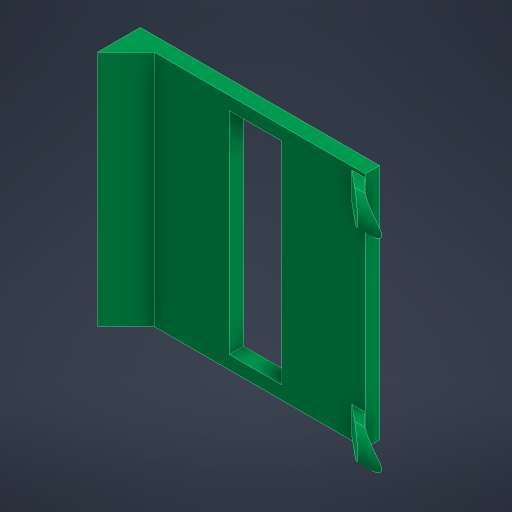
# Autodesk Inventor part: Cover Side (Normal)
Saved by Autodesk Inventor 2023.4 (Build 274418000, 418)
## iProperties
Created: 2023-02-07
Part Number: Cover Side (Normal)
Material: Generic
Document SubType Name: Modeling
Designer: xSibe
Density: 1 g/cm^3
Appearance: Plastic Dark Green
Author: xSibe
Autodesk Inventor part; units mm, degrees
ref_plane "YZ Plane" through (0, 0, 0) normal (1, 0, 0) x (0, 1, 0)
ref_plane "XZ Plane" through (0, 0, 0) normal (0, 1, 0) x (-1, 0, 0)
ref_plane "XY Plane" through (0, 0, 0) normal (0, 0, 1) x (1, 0, 0)
sketch "Sketch1" plane through (0, 0, 0) normal (0, 1, 0) x (-1, 0, 0)
  line L0 (-42.1, -24.9) -> (-7.7, -24.9)
  line L1 (-7.7, -22.55) -> (-7.7, -24.9)
  line L2 (-7.7, -22.55) -> (-42.1, -22.55)
  line L3 (-42.1, -22.55) -> (-42.1, -24.9)
  line L4 (-7.85, -24.75) -> (-41.95, -24.75)
  line L5 (-41.95, -24.75) -> (-41.95, -22.7)
  line L6 (-41.95, -22.7) -> (-7.85, -22.7)
  line L7 (-7.85, -22.7) -> (-7.85, -24.75)
  line L8 (-7.85, -22.7) -> (-11.85, -22.7)
  line L9 (-11.85, -22.7) -> (-11.85, -22.7)
  line L10 (-7.85, -18.7) -> (-7.85, -18.7)
  line L11 (-7.85, -18.7) -> (-7.85, -22.7)
  line L12 (-11.85, -22.7) -> (-7.85, -18.7)
  line L13 (0, -22.875) -> (0, -18.725)
  line L14 (-7.7, -22.875) -> (-7.7, -18.725)
  line L15 (-41.95, -22.7) -> (-39.95, -22.7)
  line L16 (-39.95, -22.7) -> (-39.95, -22.7)
  line L17 (-41.95, -20.7) -> (-41.95, -20.7)
  line L18 (-41.95, -20.7) -> (-41.95, -22.7)
  line L19 (-39.95, -22.7) -> (-41.95, -20.7)
  line L20 (-41.95, -20.7) -> (-44.07132, -18.57868)
  line L21 (-44.07132, -18.57868) -> (-45.97132, -18.57868)
  line L22 (-45.97132, -18.57868) -> (-41.95, -22.6)
  line L23 (-41.95, -22.6) -> (-39.8, -24.75)
  line L24 (-45.97132, -18.57868) -> (-45.02132, -17.62868)
  line L25 (-45.97132, -18.57868) -> (-44.198589, -18.57868) construction
  line L26 (-44.07132, -18.57868) -> (-45.02132, -17.62868)
  line L27 (-41.85, -24.825) -> (-41.85, -22.518934)
  point P0 (0, 0)
  point P1 (-11.85, -18.7)
  point P2 (-39.95, -20.7)
  point P3 (-7.85, -18.7)
  point P4 (-39.95, -22.7)
  point P5 (-41.95, -22.55)
  point P6 (-42, -22.55)
  point P7 (-41.85, -22.7)
  point P8 (-41.85, -24.75)
  dimension "d0" = 0.15
  dimension "d1" = 4
  dimension "d2" = 4
  dimension "d3" = 4
  dimension "d4" = 4
  dimension "d5" = 2
  dimension "d6" = 2
  dimension "d7" = 2
  dimension "d8" = 2
  dimension "d9" = 3
  dimension "d10" = 1.9
  dimension "d11" = 45
  dimension "d28" = 45
  constraints: 44 end point, 9 point on line, 4 horizontal, 4 parallel, 3 perpendicular, 1 collinear, 1 vertical, 5 other
  measures "d0" distance between parallel lines of L0 L4
  measures "d1" distance of point (-11.85, -18.7) L10.end
  measures "d2" distance of L8.end point (-11.85, -18.7)
  measures "d3" distance of L9.end point (-11.85, -18.7)
  measures "d4" distance of L10.start point (-11.85, -18.7)
  measures "d5" distance of L17.end point (-39.95, -20.7)
  measures "d6" distance of point (-39.95, -20.7) L15.end
  measures "d7" distance of L16.end point (-39.95, -20.7)
  measures "d8" distance of L17.start point (-39.95, -20.7)
  measures "d9" distance of L20.start L20.end
  measures "d10" distance of L20.end L21.end
  measures "d11" angle of L22 L21
  measures "d28" angle of L25 L24
extrude "Extrusion1" add sketch "Sketch1" along normal mid plane 33.75 contours L22 L21 L20 L18 L2 | L2 L18 L22 | L18 L19 L2 | L2 L27 L23 L18 | L24 L26 L21 | L11 L6 L12 L2 | L2 L12 L11 | L2 L19 L6 L27 | L6 L7 L4 L23 | L23 L4 L27
sketch "Sketch2" plane through (0, 0, 0) normal (0, 1, 0) x (-1, 0, 0)
  line L0 (-7.85, -24.75) -> (-41.85, -24.75)
  line L1 (-41.85, -22.7) -> (-45.97132, -18.57868)
  line L2 (-39.95, -22.7) -> (-11.85, -22.7)
  line L3 (-11.85, -22.7) -> (-7.85, -18.7)
  line L4 (-7.85, -18.7) -> (-7.85, -24.75)
  line L5 (-49.8, -18.72125) -> (-49.8, -22.87875)
  line L6 (-42.1, -22.55) -> (-45.92875, -18.72125)
  line L7 (0, -22.875) -> (0, -18.725)
  line L8 (-7.7, -22.875) -> (-7.7, -18.725)
  line L9 (-7.7, -18.725) -> (-7.85, -18.725)
  line L10 (-7.85, -18.725) -> (-7.85, -22.875)
  line L11 (-7.85, -22.875) -> (-7.7, -22.875)
  line L12 (-7.7, -22.875) -> (-7.7, -18.725)
  line L13 (-7.85, -18.725) -> (-6.35, -18.725)
  line L14 (-6.35, -18.725) -> (-6.35, -22.875)
  line L15 (-6.35, -22.875) -> (-7.85, -22.875)
  line L16 (-7.85, -22.875) -> (-7.85, -18.725)
  line L17 (-7.85, -22.725) -> (-6.5, -22.725)
  line L18 (-6.5, -22.725) -> (-6.5, -18.875)
  line L19 (-6.5, -18.875) -> (-7.85, -18.875)
  line L20 (-42.1, -22.87875) -> (-42.1, -22.55)
  line L21 (-42.1, -22.87875) -> (-41.67125, -22.87875)
  line L22 (-41.67125, -22.87875) -> (-42.67125, -22.87875)
  line L23 (-45.92875, -18.72125) -> (-45.82875, -18.72125)
  line L24 (-45.82875, -18.72125) -> (-48.32875, -18.72125)
  line L25 (-48.32875, -18.72125) -> (-42.67125, -22.87875)
  line L26 (-45.82875, -18.79625) -> (-48.100037, -18.79625)
  line L27 (-48.100037, -18.79625) -> (-42.646656, -22.80375)
  line L28 (-42.646656, -22.80375) -> (-41.67125, -22.80375)
  line L29 (-45.82875, -18.79625) -> (-45.75375, -18.79625)
  line L30 (-45.97132, -18.57868) -> (-45.02132, -17.62868)
  line L31 (-45.02132, -17.62868) -> (-39.95, -22.7)
  line L32 (-41.85, -24.75) -> (-41.85, -22.7)
  point P0 (0, 0)
  point P1 (-7.85, -18.875)
  point P2 (-41.74625, -22.80375)
  point P3 (-41.85, -22.80375)
  dimension "d17" = 1.5
  dimension "d18" = 0.15
  dimension "d22" = 1
  dimension "d23" = 2.5
  dimension "d24" = 0.075
  constraints: 42 end point, 8 point on line, 5 horizontal, 5 parallel, 3 perpendicular, 1 vertical, 6 other
  measures "d17" distance of L10.end L14.end
  measures "d18" distance between parallel lines of L14 L18
  measures "d22" distance of L21.end L22.end
  measures "d23" distance of L23.end L24.end
  measures "d24" distance between parallel lines of L24 L26
ref_plane "Work Plane2" through (0, -14.4, -20.8) normal (0, -1, 0) x (0, 0, -1)
ref_plane "Work Plane1" through (0, -24.9, 24.9) normal (0, -1, 0) x (0, 0, -1)
extrude "Extrusion2" add sketch "Sketch2" along normal mid plane 4 from surface at -14.4 contours L4 L19 L8 L17 | L28 L20 L6 L26 L29 L1 L32 | L8 L19 L18 L17 | L28 L27 L26 L6 L20
fillet "Fillet1" radius 2 10 edges at (7.175, -12.4, -18.875) (7.175, -16.4, -18.875) (7.175, -16.4, -22.725) (7.175, -12.4, -22.725) (45.7912, -12.4, -18.7963) (46.9644, -12.4, -18.7962) (46.9644, -16.4, -18.7962) (45.7912, -16.4, -18.7963) (42.2483, -16.4, -22.8038) (42.2483, -12.4, -22.8038)
sketch "Sketch3" plane through (46.04632, 0, -18.50368) normal (0, 1, 0) x (0.7071068, 0, -0.7071068)
  line L0 (0, 5.934493) -> (0, 0.106066)
  line L1 (0, 0.106066) -> (-1.343503, 0.106066)
  line L2 (-1.343503, 0.106066) -> (-1.343503, 7.277996)
  line L3 (-1.343503, 7.277996) -> (-21.213203, 27.147697)
  line L4 (-21.213203, 27.147697) -> (-26.870058, 27.147697)
  line L5 (-26.870058, 27.147697) -> (-22.592062, 31.425693)
  line L6 (-22.592062, 31.425693) -> (1.449569, 7.384062)
  line L7 (1.148836, 2.093348) -> (1.148836, 2.093348)
  line L8 (1.148836, 2.093348) -> (0, 3.242184)
  line L9 (0, 3.242184) -> (0, 3.242184)
  line L10 (0, 3.242184) -> (1.148836, 2.093348)
  line L11 (1.146923, 2.105868) -> (1.146923, 2.105868)
  line L12 (1.146923, 2.105868) -> (0, 3.252791)
  line L13 (0, 3.252791) -> (0, 5.934493)
  line L14 (0, 3.252791) -> (1.146923, 2.105868)
  line L15 (1.146923, 2.105868) -> (0, 3.252791)
  line L16 (1.148836, 2.093348) -> (1.146923, 2.105868)
  line L17 (0, 3.242184) -> (1.148836, 2.093348)
  line L18 (0, 3.252791) -> (0, 3.242184)
  line L19 (-25.3321, 28.685654) -> (-25.3321, 28.685654)
  line L20 (-24.023953, 30.099867) -> (-26.039207, 30.099867)
  line L21 (-24.023953, 30.099867) -> (-22.008699, 30.099867) construction
  line L22 (-26.85238, 27.27144) -> (-26.85238, 29.286695)
  line L23 (-26.85238, 27.27144) -> (-24.837126, 27.27144) construction
  line L24 (-27.860007, 28.279067) -> (-26.85238, 27.27144)
  line L25 (-25.03158, 31.107495) -> (-24.023953, 30.099867)
  line L26 (0.636683, 5.444535) -> (0.073362, 6.007855)
  line L27 (0.073362, 6.007855) -> (0.829619, 4.18209)
  line L28 (0.073362, 6.007855) -> (2.049557, 6.007855) construction
  line L29 (0.636683, 5.444535) -> (1.146923, 2.105868)
  line L30 (1.148836, 2.093348) -> (1.659075, -1.245318)
  line L31 (1.659075, -1.245318) -> (0.073362, 6.007855)
  line L32 (0, 0.413757) -> (0, 3.242184)
  line L33 (0, 0.413757) -> (-1.343503, 7.277996)
  line L34 (-0.671751, 0.106066) -> (-1.343503, 7.277996)
  line L35 (-26.286695, 29.640248) -> (-26.286695, 29.640248)
  line L36 (-26.286695, 29.640248) -> (-25.3321, 28.685654)
  line L37 (-25.3321, 28.685654) -> (-26.286695, 29.640248)
  line L38 (-27.700908, 28.226034) -> (-26.746314, 27.27144)
  line L39 (-27.700908, 28.226034) -> (-26.286695, 29.640248)
  line L40 (-26.286695, 29.640248) -> (-24.978547, 30.948396)
  line L41 (-24.978547, 30.948396) -> (-24.023953, 29.993801)
  line L42 (0, 5.934493) -> (1.659075, -1.245318)
  line L43 (0, 5.934493) -> (0, 5.934493)
  line L44 (0, 3.252791) -> (0, 5.934493)
  line L45 (1.449569, 7.384062) -> (0, 5.934493)
  point P0 (0.864735, 2.388056)
  point P1 (0.867703, 2.374481)
  point P2 (1.146923, 2.105868)
  point P3 (-24.130019, 30.099867)
  point P4 (-25.827075, 30.099867)
  point P5 (-26.85238, 29.074563)
  point P6 (-26.85238, 27.377506)
  dimension "d37" = 180
  dimension "d38" = 90
  dimension "d39" = 67.5
  constraints: 24 end point, 3 equal length, 3 horizontal, 1 midpoint, 1 perpendicular, 1 point on line, 1 other
  measures "d37" angle of L20 L21
  measures "d38" angle of L23 L22
  measures "d39" angle of L27 L28
extrude "Extrusion3" cut sketch "Sketch3" along normal mid plane 5 from surface at -14.4 contours L26 L29 L27 | L27 L29 L12 L31 | L12 L16 L8 L31 | L8 L30 L31
mirror "Mirror1" about plane through (0, 0, 0) normal (0, 1, 0) of "Extrusion2", "Fillet1", "Extrusion3"
extrude "Extrusion5" cut sketch "Sketch3" along normal mid plane 50 contours L34 L1 L2
sketch "Sketch5" plane through (41.95, 16.875, -24.75) normal (0, 0, -1) x (-1, 0, 0)
  line L0 (34.1, -33.75) -> (34.1, 0) projected
  line L1 (0.1, 0) -> (34.1, 0) projected
  line L2 (34.1, -33.75) -> (0.1, -33.75) projected
  line L3 (34.1, -16.875) -> (15.7, -16.875)
  line L4 (19.45, -31.875) -> (11.95, -31.875)
  line L5 (11.95, -31.875) -> (11.95, -1.875)
  line L6 (11.95, -1.875) -> (19.45, -1.875)
  line L7 (19.45, -1.875) -> (19.45, -31.875)
  line L8 (19.45, -31.875) -> (11.95, -1.875) construction
  line L9 (11.95, -31.875) -> (19.45, -1.875) construction
  line L10 (0.1, -33.75) -> (0.1, 0) projected
  point P0 (41.95, -16.875)
  dimension "d42" = 18.4
  dimension "d43" = 7.5
  dimension "d44" = 30
  constraints: 14 end point, 3 midpoint, 2 horizontal, 2 parallel, 1 perpendicular
  measures "d42" distance of L3.start L3.end
  measures "d43" distance of L5.end L6.end
  measures "d44" distance of L4.end L5.end
extrude "Extrusion6" cut sketch "Sketch5" against normal up to surface (2.05 mm away) contours L4 L5 L6 L7
sketch "Sketch6" plane through (41.85, 0, 0) normal (1, 0, 0) x (0, 1, 0)
  arc A0 (13.764204, -22.7) -> (14.4, -22.80375) centre (14.4, -20.80375) ccw
  line L0 (-13.764204, -22.7) -> (13.764204, -22.7)
  arc A1 (-14.4, -22.80375) -> (-13.764204, -22.7) centre (-14.4, -20.80375) ccw
  arc A2 (-15.035796, -22.7) -> (-14.4, -22.80375) centre (-14.4, -20.80375) ccw
  line L1 (-15.035796, -22.7) -> (-16.875, -22.7)
  line L2 (-16.875, -24.75) -> (-16.875, -22.7)
  line L3 (-16.875, -24.75) -> (16.875, -24.75)
  line L4 (16.875, -22.7) -> (16.875, -24.75)
  line L5 (15.035796, -22.7) -> (16.875, -22.7)
  arc A3 (14.4, -22.80375) -> (15.035796, -22.7) centre (14.4, -20.80375) ccw
  line L6 (16.875, -18.10368) -> (-16.875, -18.10368)
  arc A4 (16.4, -20.79625) -> (12.4, -20.79625) centre (14.4, -20.79625) ccw
  line L7 (12.4, -20.80375) -> (12.4, -20.79625)
  arc A5 (12.4, -20.80375) -> (14.4, -22.80375) centre (14.4, -20.80375) ccw
  arc A6 (14.4, -22.80375) -> (16.4, -20.80375) centre (14.4, -20.80375) ccw
  line L8 (16.4, -20.79625) -> (16.4, -20.80375)
  arc A7 (-12.4, -20.79625) -> (-16.4, -20.79625) centre (-14.4, -20.79625) ccw
  line L9 (-16.4, -20.80375) -> (-16.4, -20.79625)
  arc A8 (-16.4, -20.80375) -> (-14.4, -22.80375) centre (-14.4, -20.80375) ccw
  arc A9 (-14.4, -22.80375) -> (-12.4, -20.80375) centre (-14.4, -20.80375) ccw
  line L10 (-12.4, -20.79625) -> (-12.4, -20.80375)
  line L11 (14.4, -18.79625) -> (-14.4, -18.79625)
  line L12 (-16.875, -18.57868) -> (-16.875, -18.10368)
  line L13 (-16.875, -22.7) -> (-16.875, -18.57868)
  line L14 (16.875, -18.10368) -> (16.875, -18.57868)
  line L15 (16.875, -18.57868) -> (16.875, -22.7)
  line L16 (16.4, -20.80375) -> (16.4, -22.7)
  line L17 (-16.4, -20.80375) -> (-16.4, -22.7)
  line L18 (12.4, -20.80375) -> (12.4, -22.7)
  line L19 (-12.4, -20.80375) -> (-12.4, -22.7)
  point P0 (-15.035796, -22.7)
  point P1 (13.764204, -22.7)
  point P2 (13.764204, -22.7)
  point P3 (-15.035796, -22.7)
  constraints: 10 end point, 4 point on line, 4 tangent, 3 perpendicular, 2 point on circle, 1 vertical
extrude "Extrusion7" cut sketch "Sketch6" along normal mid plane 33.75 contours L0 L19 L10 A7 L11 A4 L7 L18 | L16 L8 A4 L11 A7 L9 L17 L1 L13 L12 L6 L14 L15 L5
sketch "Sketch7" plane through (0, 0, 0) normal (0, 1, 0) x (-1, 0, 0)
  line L0 (-44.980867, -20.79625) -> (-44.980867, -20.79625)
  line L1 (-44.980867, -20.79625) -> (-42.247231, -20.79625)
  line L2 (-42.247231, -20.79625) -> (-44.980867, -20.79625)
  line L3 (-41.85, -22.80375) -> (-44.96917, -20.80375)
  line L4 (-44.96917, -20.80375) -> (-43.74625, -20.80375)
  line L5 (-43.74625, -20.80375) -> (-41.85, -22.7)
  line L6 (-41.85, -22.80375) -> (-41.85, -22.7)
  line L7 (-44.96917, -20.80375) -> (-44.980867, -20.79625)
  line L8 (-42.247231, -20.79625) -> (-44.980867, -20.79625)
  line L9 (-43.74625, -20.80375) -> (-41.85, -22.7)
  line L10 (-44.96917, -20.80375) -> (-43.74625, -20.80375)
  line L11 (-44.660605, -18.79625) -> (-48.100037, -18.79625)
  line L12 (-44.980867, -20.79625) -> (-48.100037, -18.79625)
  line L13 (-42.247231, -20.79625) -> (-44.660605, -18.79625)
  line L14 (-41.85, -22.7) -> (-11.85, -22.7)
  line L15 (-11.85, -22.7) -> (-7.85, -18.7)
  line L16 (-7.85, -18.7) -> (-7.85, -24.75)
  line L17 (-7.85, -24.75) -> (-41.85, -24.75)
  line L18 (-41.85, -24.75) -> (-41.85, -22.7)
  line L19 (-41.85, -24.75) -> (-41.825, -24.75)
  line L20 (-41.825, -24.75) -> (-41.825, -22.7)
  line L21 (-41.825, -22.7) -> (-41.85, -22.7)
  line L22 (-41.85, -22.7) -> (-41.85, -24.75)
  arc A0 (-41.825, -22.7) -> (-48.100037, -18.79625) centre (-50.363142, -29.429293) ccw
  line L23 (-39.95, -22.7) -> (-42.247231, -20.79625)
  line L24 (-39.95, -22.7) -> (-41.85, -22.7)
  line L25 (-42.247231, -20.79625) -> (-42.247231, -20.79625)
  point P0 (0, 0)
  point P1 (-41.85, -22.80375)
  dimension "d54" = 0.025
  constraints: 8 end point, 3 point on circle, 2 parallel, 1 centre point, 1 horizontal, 1 perpendicular, 1 point on line
  measures "d54" distance of L21.end L20.end
extrude "Extrusion8" cut sketch "Sketch7" along normal mid plane 40 contours L12 A0 L1 | L1 A0 L4 L7 | L4 L5 L6 L3 | A0 L14 L5 | L6 L14 L20 L17 L18
sketch "Sketch8" plane through (7.85, -16.875, -18.7) normal (-1, 0, 0) x (0, 0, 1)
  line L0 (-4.025, 31.269367) -> (-4.025, 31.280633)
  arc A0 (-2.175, 33.275) -> (-4.025, 31.280633) centre (-2.025, 31.280633) ccw
  arc A1 (-2.175, 29.275) -> (-2.175, 33.275) centre (-2.175, 31.275) ccw
  arc A2 (-4.025, 31.269367) -> (-2.175, 29.275) centre (-2.025, 31.269367) ccw
  line L1 (-4.025, 2.469367) -> (-4.025, 2.480633)
  arc A3 (-2.175, 4.475) -> (-4.025, 2.480633) centre (-2.025, 2.480633) ccw
  arc A4 (-2.175, 0.475) -> (-2.175, 4.475) centre (-2.175, 2.475) ccw
  arc A5 (-4.025, 2.469367) -> (-2.175, 0.475) centre (-2.025, 2.469367) ccw
  line L2 (0, 0) -> (0, 33.75)
  line L3 (-6.05, 33.75) -> (0, 33.75)
  line L4 (-6.05, 0) -> (-6.05, 33.75)
  line L5 (0, 0) -> (-6.05, 0)
  arc A6 (-2.169367, 29.425009) -> (-2.169367, 33.124991) centre (-2.175, 31.275) ccw
  arc A7 (-2.169367, 33.124991) -> (-3.875, 31.280633) centre (-2.025, 31.280633) ccw
  line L6 (-3.875, 31.280633) -> (-3.875, 31.269367)
  arc A8 (-3.875, 31.269367) -> (-2.169367, 29.425009) centre (-2.025, 31.269367) ccw
  line L7 (-3.875, 2.480633) -> (-3.875, 2.469367)
  arc A9 (-3.875, 2.469367) -> (-2.169367, 0.625009) centre (-2.025, 2.469367) ccw
  arc A10 (-2.169367, 0.625009) -> (-2.169367, 4.324991) centre (-2.175, 2.475) ccw
  arc A11 (-2.169367, 4.324991) -> (-3.875, 2.480633) centre (-2.025, 2.480633) ccw
  point P0 (18.7, 16.875)
  dimension "d55" = 0.15
  dimension "d56" = 0.15
  constraints: 12 point on circle, 6 centre point, 4 end point, 6 other
  measures "d55" radial gap between concentric circles of A2 A8
  measures "d56" radial gap between concentric circles of A3 A11
extrude "Extrusion9" cut sketch "Sketch8" along normal blind 10 contours L0 A0 A1 A2 | L1 A3 A4 A5
chamfer "Chamfer2" distance 1.35 angle 45 8 edges at (6.5, -14.4, -19.025) (6.5, -15.6617, -22.0832) (6.5, -14.4, -22.575) (6.5, -13.1383, -22.0832) (6.5, 14.4, -19.025) (6.5, 13.1383, -22.0832) (6.5, 14.4, -22.575) (6.5, 15.6617, -22.0832)
equation "\"d4\" = d3"
equation "\"d8\" = d7"
body "Solid1"
